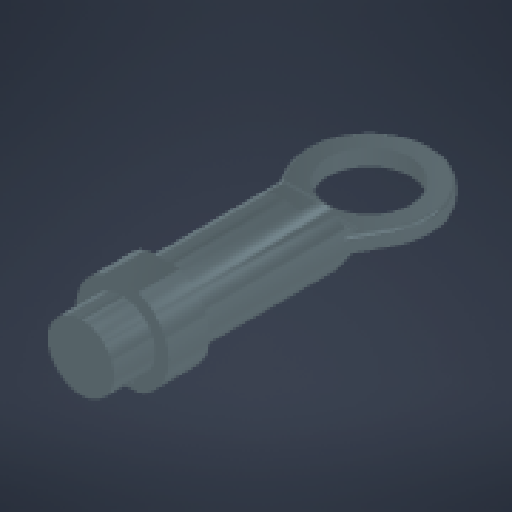
# Autodesk Inventor part: vòng bi_dài 35mm
Saved by Autodesk Inventor 2027.1 (Build 311270010, 270A)
## iProperties
Created: 2026-08-09
Part Number: vòng bi_dài 35mm
Material: Generic
Document SubType Name: Sheet Metal
Designer: MSI
Density: 1 g/cm^3
Sheet Metal Rule: Default_mm
Appearance: Lead
Author: MSI
Autodesk Inventor part; units mm, degrees
ref_plane "YZ Plane" through (0, 0, 0) normal (1, 0, 0) x (0, 1, 0)
ref_plane "XZ Plane" through (0, 0, 0) normal (0, 1, 0) x (-1, 0, 0)
ref_plane "XY Plane" through (0, 0, 0) normal (0, 0, 1) x (1, 0, 0)
sketch "Sketch1" plane through (0, 0, 0) normal (0, 0, 1) x (1, 0, 0)
  circle A0 centre (0, 0) radius 4
  line L0 (-1.555751, 4.751804) -> (1.555751, 4.751804)
  line L1 (0, 0) -> (1.555751, 0)
  line L2 (-1.555751, -4.751804) -> (1.555751, -4.751804)
  arc A1 (-1.555751, 4.751804) -> (-1.555751, -4.751804) centre (0, 0) ccw
  arc A2 (1.555751, -4.751804) -> (1.555751, 4.751804) centre (0, 0) ccw
  circle A3 centre (0, 0) radius 4.5
  dimension "d0" = 8
  dimension "d2" = 9
  constraints: 6 end point, 4 centre point, 4 point on circle, 3 coincident, 2 horizontal, 2 symmetric about line
  measures "d0" diameter of A0
  measures "d2" diameter of A3
extrude "Extrusion1" add sketch "Sketch1" along normal blind 27.5 contours A0
extrude "Extrusion2" add sketch "Sketch1" along normal blind 22.5 contours A3
sketch "Sketch2" plane through (0, 0, 22.5) normal (0, 0, 1) x (1, 0, 0)
  circle A0 centre (0, 0) radius 5.629087
  line L0 (0, 0) -> (1.158118, 0)
  line L1 (-1.971905, 5.2724) -> (1.971905, 5.2724)
  line L2 (-1.971905, -5.2724) -> (1.971905, -5.2724)
  constraints: 6 end point, 2 horizontal, 2 point on circle, 2 symmetric about line, 1 centre point, 1 coincident
extrude "Extrusion3" add sketch "Sketch2" against normal blind 5 contours A0 L2 L1
sketch "Sketch3" plane through (0, 0, 0) normal (0, 0, -1) x (-1, 0, 0)
  circle A0 centre (0, 0) radius 4.5
  line L0 (-2.019433, 4.021429) -> (2.019433, 4.021429)
  line L1 (0, 0) -> (1.467716, 0)
  line L2 (-2.019433, -4.021429) -> (2.019433, -4.021429)
  arc A1 (2.019433, 4.021429) -> (-2.019433, 4.021429) centre (0, 0) ccw
  arc A2 (-2.019433, -4.021429) -> (2.019433, -4.021429) centre (0, 0) ccw
  constraints: 6 end point, 6 point on circle, 2 centre point, 2 horizontal, 2 symmetric about line, 1 coincident
extrude "Extrusion4" cut sketch "Sketch3" against normal blind 3 contours L0 A0 | A0 L2
sketch "Sketch4" plane through (0, 0, 0) normal (0, 1, 0) x (-1, 0, 0)
  circle A0 centre (0, -7.5) radius 7.5
  line L0 (2.019433, 0) -> (-2.019433, 0)
  line L1 (-2.019433, 0) -> (-4.5, 0)
  line L2 (-4.5, 0) -> (4.599623, 0)
  arc A1 (-4.5, 0) -> (-6.78711, -4.308583) centre (38.772452, -25.731481) ccw
  line L3 (4.599623, 0) -> (6.684935, -4.099757)
  line L4 (-4.5, 0) -> (4.599623, 0)
  point P0 (0, 0)
  point P1 (0, 0)
  dimension "d11" = 15
  dimension "d12" = 7.5
  constraints: 6 end point, 4 point on circle, 2 centre point, 2 tangent, 1 collinear, 1 horizontal, 1 midpoint
  measures "d11" diameter of A0
  measures "d12" distance of point (0, 0) A0.centre
extrude "Extrusion5" add sketch "Sketch4" against normal blind 1
extrude "Extrusion6" add sketch "Sketch4" along normal blind 1
sketch "Sketch6" plane through (0, 1, 0) normal (0, 1, 0) x (1, 0, 0)
  arc A0 (6.78711, 4.308583) -> (-6.684935, 4.099757) centre (0, 7.5) ccw
  circle A1 centre (0, 7.5) radius 5
  point P0 (0, 0)
  dimension "d17" = 10
  constraints: 1 centre point, 1 coincident
  measures "d17" diameter of A1
extrude "Extrusion7" cut sketch "Sketch6" against normal blind 2
fillet "Fillet1" radius 2 2 edges at (0, 1, 0) (0, -1, 0)
fillet "Fillet2" radius 1 2 edges at (0, -4.0214, 0) (0, 4.0214, 0)
fillet "Fillet3" radius 0.5 6 edges at (-5.6423, 1, -2.0499) (5.6958, 1, -2.1266) (-0.1162, 1, -14.9991) (5.6958, -1, -2.1266) (-5.6423, -1, -2.0499) (-0.1162, -1, -14.9991)
equation "\"BendRadius\" = Thickness"
equation "\"BendReliefWidth\" = Thickness"
equation "\"BendReliefDepth\" = 0.5 * Thickness"
equation "\"CornerReliefSize\" = 4 * Thickness"
equation "\"MinimumRemnant\" = 2 * Thickness"
equation "\"TransitionRadius\" = BendRadius"
equation "\"JacobiRadiusSize\" = BendRadius"
equation "\"GapSize\" = Thickness"
equation "\"Thickness\" = 0.5"
body "Solid1"
